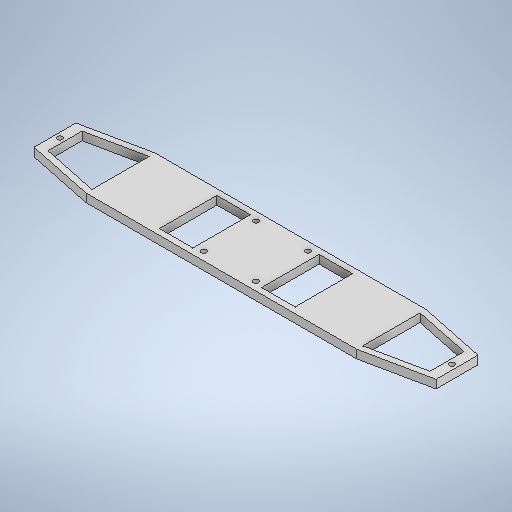
# Autodesk Inventor part: nakladka
Saved by Autodesk Inventor 2025.3 (Build 293356000, 356)
## iProperties
Created: 2026-04-12
Part Number: nakladka
Material: Generic
Document SubType Name: Modeling
Designer: ksawe
Density: 1 g/cm^3
Appearance: Default
Author: ksawe
Autodesk Inventor part; units mm, degrees
ref_plane "YZ Plane" through (0, 0, 0) normal (1, 0, 0) x (0, 1, 0)
ref_plane "XZ Plane" through (0, 0, 0) normal (0, 1, 0) x (-1, 0, 0)
ref_plane "XY Plane" through (0, 0, 0) normal (0, 0, 1) x (1, 0, 0)
sketch "Sketch1" plane through (0, 0, 0) normal (0, 1, 0) x (-1, 0, 0)
  line L0 (-120, 12.5) -> (-120, -12.5)
  line L1 (-120, 12.5) -> (-80.837, 20.64)
  line L2 (-80.837, 20.64) -> (0, 20.64)
  line L3 (-120, 0) -> (120, 0) construction
  line L4 (-120, -12.5) -> (-80.837, -20.64)
  line L5 (-80.837, -20.64) -> (0, -20.64)
  line L6 (0, 20.64) -> (0, -20.64) construction
  line L7 (80.837, 20.64) -> (0, 20.64)
  line L8 (120, 12.5) -> (80.837, 20.64)
  line L9 (120, -12.5) -> (80.837, -20.64)
  line L10 (120, 12.5) -> (120, -12.5)
  line L11 (80.837, -20.64) -> (0, -20.64)
  line L12 (-80.837, -17.0652) -> (-114, -10.1723)
  line L13 (-80.837, 17.0652) -> (-114, 10.1723)
  line L14 (-114, 10.1723) -> (-114, -10.1723)
  line L15 (-80.837, 17.0652) -> (-80.837, -17.0652)
  line L16 (-20.5, 17.14) -> (-40.5, 17.14)
  line L17 (-40.5, 17.14) -> (-40.5, -17.14)
  line L18 (-40.5, -17.14) -> (-20.5, -17.14)
  line L19 (-20.5, -17.14) -> (-20.5, 17.14)
  line L20 (80.837, -17.0652) -> (114, -10.1723)
  line L21 (80.837, 17.0652) -> (114, 10.1723)
  line L22 (114, 10.1723) -> (114, -10.1723)
  line L23 (80.837, 17.0652) -> (80.837, -17.0652)
  line L24 (20.5, 17.14) -> (40.5, 17.14)
  line L25 (40.5, 17.14) -> (40.5, -17.14)
  line L26 (40.5, -17.14) -> (20.5, -17.14)
  line L27 (20.5, -17.14) -> (20.5, 17.14)
  circle A0 centre (-117, 0) radius 1.5
  circle A1 centre (-15.5, -15.64) radius 1.5
  circle A2 centre (15.5, -15.64) radius 1.5
  circle A3 centre (-15.5, 15.64) radius 1.5
  circle A4 centre (15.5, 15.64) radius 1.5
  circle A5 centre (117, 0) radius 1.5
  point P0 (0, 0)
  point P1 (0, 0)
  point P2 (0, 0)
  point P3 (0, 0)
  point P4 (-114, 0)
  point P5 (-30.5, 17.14)
  dimension "d0" = 25
  dimension "d1" = 40
  dimension "d2" = 80.837
  dimension "d3" = 39.163
  dimension "d6" = 3.5
  dimension "d7" = 6
  dimension "d8" = 93.5
  dimension "d9" = 3.5
  dimension "d10" = 3.5
  dimension "d11" = 20
  dimension "d12" = 3
  dimension "d13" = 3
  dimension "d14" = 5
  dimension "d15" = 5
  dimension "d16" = 3
  constraints: 56 end point, 20 symmetric about line, 6 centre point, 6 midpoint, 4 vertical, 3 coincident, 3 horizontal, 3 parallel, 1 perpendicular, 1 point on line, 1 vertical alignment, 4 other
  measures "d0" distance of L0.start L0.end
  measures "d1" distance of L0.start L1.end
  measures "d2" distance of L1.end L2.end
  measures "d3" horizontal distance of L0.end L4.end
  measures "d6" distance between parallel lines of L4 L12
  measures "d7" distance between parallel lines of L0 L14
  measures "d8" distance from line of point (-114, 0) L19
  measures "d9" distance from line of L2 point (-30.5, 17.14)
  measures "d10" distance between parallel lines of L5 L18
  measures "d11" distance of L16.start L16.end
  measures "d12" diameter of A0
  measures "d13" diameter of A1
  measures "d14" distance from line of L5 A1.centre
  measures "d15" distance from line of L19 A1.centre
  measures "d16" distance from line of L0 A0.centre
extrude "Extrusion1" add sketch "Sketch1" along normal mid plane 5
body "Solid1"
